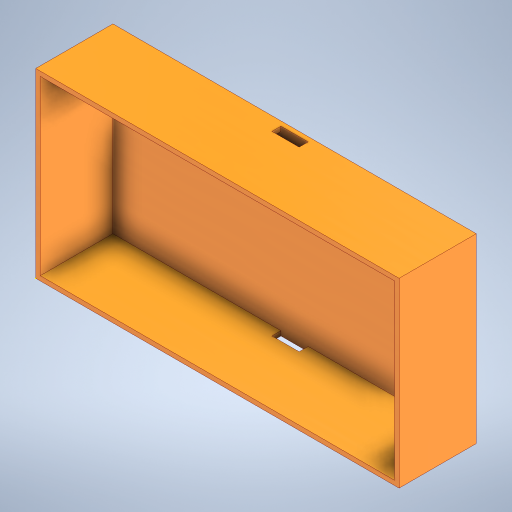
# Autodesk Inventor part: d
Saved by Autodesk Inventor 2024 (Build 280153000, 153)
## iProperties
Created: 2023-06-04
Part Number: d
Material: Generic
Document SubType Name: Modeling
Designer: hithi
Density: 1 g/cm^3
Appearance: Light Red
Author: hithi
Autodesk Inventor part; units mm, degrees
ref_plane "YZ Plane" through (0, 0, 0) normal (1, 0, 0) x (0, 1, 0)
ref_plane "XZ Plane" through (0, 0, 0) normal (0, 1, 0) x (-1, 0, 0)
ref_plane "XY Plane" through (0, 0, 0) normal (0, 0, 1) x (1, 0, 0)
sketch "Sketch1" plane through (0, 0, 0) normal (0, 0, 1) x (1, 0, 0)
  line L0 (0, 0) -> (400, 0)
  line L1 (400, 0) -> (400, 200)
  line L2 (400, 200) -> (0, 200)
  line L3 (0, 200) -> (0, 0)
  line L4 (5, 5) -> (395, 5)
  line L5 (395, 5) -> (395, 195)
  line L6 (395, 195) -> (5, 195)
  line L7 (5, 195) -> (5, 5)
  dimension "d0" = 400
  dimension "d1" = 200
  dimension "d2" = 390
  dimension "d3" = 190
  constraints: 16 end point, 4 parallel, 2 horizontal, 2 perpendicular
  measures "d0" distance of L2.end L1.end
  measures "d1" distance of L1.end L0.end
  measures "d2" distance of L6.end L5.end
  measures "d3" distance of L5.end L4.end
extrude "Extrusion1" add sketch "Sketch1" along normal blind 80
sketch "Sketch2" plane through (0, 0, 0) normal (0, -1, 0) x (1, 0, 0)
  line L0 (5, 0) -> (395, 0) projected
  line L1 (190, 0) -> (220, 0)
  line L2 (220, 0) -> (220, 10)
  line L3 (220, 10) -> (190, 10)
  line L4 (190, 10) -> (190, 0)
  point P0 (0, 0)
  dimension "d6" = 30
  dimension "d7" = 10
  constraints: 8 end point, 2 parallel, 1 horizontal, 1 perpendicular, 1 point on line
  measures "d6" distance of L3.end L2.end
  measures "d7" distance of L2.end L1.end
extrude "Extrusion2" cut sketch "Sketch2" against normal blind 80
sketch "Sketch3" plane through (0, 200, 0) normal (0, 1, 0) x (1, 0, 0)
  line L0 (190, -10) -> (220, -10) projected
  line L1 (190, 0) -> (5, 0) projected
  line L2 (220, -10) -> (190, -10)
  line L3 (190, -10) -> (190, 0)
  line L4 (190, 0) -> (220, 0)
  line L5 (220, 0) -> (220, -10)
  point P0 (0, 0)
  constraints: 8 end point, 2 parallel, 1 horizontal, 1 perpendicular
extrude "Extrusion3" cut sketch "Sketch3" against normal blind 80
sketch "Sketch4" plane through (0, 0, 0) normal (0, 0, -1) x (-1, 0, 0)
  line L0 (-400, 200) -> (-220, 200) projected
  line L1 (0, 0) -> (-400, 0)
  line L2 (-400, 0) -> (-400, 200)
  line L3 (-400, 200) -> (0, 200)
  line L4 (0, 200) -> (0, 0)
  constraints: 8 end point, 2 parallel, 1 horizontal, 1 perpendicular
extrude "Extrusion4" add sketch "Sketch4" along normal blind 5
sketch "Sketch5" plane through (0, 0, 80) normal (0, 0, 1) x (1, 0, 0)
  point P0 (0, 0)
body "Solid1"
